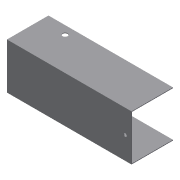
# Autodesk Inventor part: U profil
Saved by Autodesk Inventor 2015 (Build 190159000, 159)
## iProperties
Created: 2015-01-07
Part Number: U profil
Material: Všeobecné
Document SubType Name: Modeling
Designer: Michal
Density: 1 g/cm^3
Appearance: Výchozí
Author: Michal
Autodesk Inventor part; units mm, degrees
ref_plane "YZ Plane" through (0, 0, 0) normal (1, 0, 0) x (0, 1, 0)
ref_plane "XZ Plane" through (0, 0, 0) normal (0, 1, 0) x (-1, 0, 0)
ref_plane "XY Plane" through (0, 0, 0) normal (0, 0, 1) x (1, 0, 0)
sketch "Náčrt1" plane through (0, 0, 0) normal (1, 0, 0) x (0, 1, 0)
  line L0 (0, 0) -> (130, 0)
  line L1 (130, 0) -> (130, -2)
  line L2 (130, -2) -> (2, -2)
  line L3 (2, -2) -> (2, -142)
  line L4 (2, -142) -> (130, -142)
  line L5 (130, -142) -> (130, -144)
  line L6 (130, -144) -> (0, -144)
  line L7 (0, -144) -> (0, 0)
  dimension "d0" = 130
  dimension "d1" = 2
  dimension "d2" = 128
  dimension "d3" = 140
  dimension "d4" = 128
  dimension "d5" = 2
  dimension "d6" = 130
  constraints: 16 end point, 4 perpendicular, 2 point on line, 1 horizontal
  measures "d0" distance of L0.start L0.end
  measures "d1" distance of L0.end L1.end
  measures "d2" distance of L1.end L2.end
  measures "d3" distance of L2.end L3.end
  measures "d4" distance of L3.end L4.end
  measures "d5" distance of L4.end L5.end
  measures "d6" distance of L5.end L6.end
extrude "Vysunutí1" add sketch "Náčrt1" along normal blind 390
sketch "Náčrt2" plane through (0, 0, 0) normal (0, 0, 1) x (1, 0, 0)
  circle A0 centre (78, 104) radius 8
  line L0 (0, 0) -> (0, 130) projected
  line L1 (0, 0) -> (390, 0) projected
  line L2 (390, 130) -> (390, 0) projected
  line L3 (0, 130) -> (390, 130) projected
  dimension "d9" = 16
  dimension "d10" = 312
  dimension "d11" = 26
  constraints: 1 centre point
  measures "d9" diameter of A0
  measures "d10" distance from line of L2 A0.centre
  measures "d11" distance from line of L3 A0.centre
extrude "Vysunutí2" cut sketch "Náčrt2" against normal through all contours A0
sketch "Náčrt4" plane through (0, 2, -2) normal (0, 1, 0) x (1, 0, 0)
  line L0 (0, 0) -> (0, 140) projected
  line L1 (0, 0) -> (390, 0) projected
  line L2 (390, 140) -> (390, 0) projected
  line L3 (0, 140) -> (390, 140) projected
  circle A0 centre (370, 72) radius 5
  line L4 (0, 142) -> (390, 142) projected
  point P0 (0, -2)
  dimension "d14" = 20
  dimension "d15" = 70
  dimension "d16" = 10
  constraints: 1 centre point
  measures "d14" distance from line of L2 A0.centre
  measures "d15" distance from line of L4 A0.centre
  measures "d16" diameter of A0
extrude "Vysunutí3" cut sketch "Náčrt4" against normal through all contours A0
